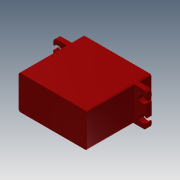
# Autodesk Inventor part: standart_servo
Saved by Autodesk Inventor 2015 (Build 190159000, 159)
## iProperties
Created: 2013-01-22
Part Number: standart_servo
Material: Generic
Document SubType Name: Modeling
Designer: idle-rug
Density: 1 g/cm^3
Appearance: Default
Author: idle-rug
Autodesk Inventor part; units mm, degrees
ref_plane "YZ Plane" through (0, 0, 0) normal (1, 0, 0) x (0, 1, 0)
ref_plane "XZ Plane" through (0, 0, 0) normal (0, 1, 0) x (-1, 0, 0)
ref_plane "XY Plane" through (0, 0, 0) normal (0, 0, 1) x (1, 0, 0)
sketch "Sketch1" plane through (0, 0, 0) normal (0, 1, 0) x (-1, 0, 0)
  line L0 (-20.1, -10) -> (20.1, -10)
  line L1 (20.1, -10) -> (20.1, 10)
  line L2 (20.1, 10) -> (-20.1, 10)
  line L3 (-20.1, 10) -> (-20.1, -10)
  line L4 (-20.1, -10) -> (20.1, 10) construction
  line L5 (20.1, -10) -> (-20.1, 10) construction
  point P0 (0, 0)
  constraints: 12 end point, 2 midpoint, 2 parallel, 1 horizontal, 1 perpendicular
extrude "Extrusion1" add sketch "Sketch1" along normal blind 43.7
sketch "Sketch2" plane through (20.1, 0, 10) normal (1, 0, 0) x (0, 0, -1)
  line L0 (20, 0) -> (20, 43.7) projected
  line L1 (0, 0) -> (0, 43.7) projected
  line L2 (20, 27.8) -> (0, 27.8)
  line L3 (0, 27.8) -> (0, 30.6)
  line L4 (0, 30.6) -> (20, 30.6)
  line L5 (20, 30.6) -> (20, 27.8)
  point P0 (10, 0)
  constraints: 8 end point, 4 point on line, 2 perpendicular, 1 collinear
sketch "Sketch3" plane through (-20.1, 0, -10) normal (-1, 0, 0) x (0, 0, 1)
  line L0 (20, 0) -> (20, 43.7) projected
  line L1 (0, 0) -> (0, 43.7) projected
  line L2 (20, 27.8) -> (0, 27.8)
  line L3 (0, 27.8) -> (0, 30.6)
  line L4 (0, 30.6) -> (20, 30.6)
  line L5 (20, 30.6) -> (20, 27.8)
  point P0 (10, 0)
  constraints: 8 end point, 4 point on line, 2 perpendicular
extrude "Extrusion2" add sketch "Sketch3" along normal blind 7.4
extrude "Extrusion3" add sketch "Sketch2" along normal blind 7.4
sketch "Sketch4" plane through (0, 43.7, 0) normal (0, 1, 0) x (1, 0, 0)
  line L0 (20.1, 10) -> (-20.1, 10) projected
  line L1 (-20.1, 10) -> (-20.1, -10) projected
  line L2 (-20.1, -10) -> (20.1, -10) projected
  line L3 (20.1, -10) -> (20.1, 10) projected
  circle A0 centre (-9.4, 0) radius 6.8
  circle A1 centre (-9.4, 0) radius 5.1
  circle A2 centre (-9.4, 0) radius 3
  constraints: 3 centre point, 2 coincident
extrude "Extrusion4" cut sketch "Sketch4" against normal blind 5.8 contours L3 L2 L1 L0
sketch "Sketch5" plane through (-9.4, 43.7, 0) normal (0, 1, 0) x (1, 0, 0)
  circle A0 centre (0, 0) radius 6.8 projected
  circle A1 centre (0, 0) radius 2.5
  dimension "d20" = 5
  constraints: 1 centre point, 1 coincident
  measures "d20" diameter of A1
extrude "Extrusion5" cut sketch "Sketch5" against normal blind 4
fillet "Fillet1" radius 2 1 edges at (-27.5, 29.2, 10)
fillet "Fillet2" radius 2 1 edges at (27.5, 29.2, 10)
fillet "Fillet3" radius 2 1 edges at (27.5, 29.2, -10)
fillet "Fillet4" radius 2 1 edges at (-27.5, 29.2, -10)
fillet "Fillet5" radius 1 1 edges at (-20.1, 34.25, -10)
fillet "Fillet6" radius 1 1 edges at (-20.1, 13.9, -10)
fillet "Fillet7" radius 1 1 edges at (-20.1, 34.25, 10)
fillet "Fillet8" radius 1 1 edges at (-20.1, 13.9, 10)
fillet "Fillet9" radius 1 1 edges at (20.1, 34.25, 10)
fillet "Fillet10" radius 1 1 edges at (20.1, 13.9, 10)
fillet "Fillet11" radius 1 1 edges at (20.1, 34.25, -10)
fillet "Fillet12" radius 1 1 edges at (20.1, 13.9, -10)
sketch "Sketch6" plane through (-9.4, 43.7, 0) normal (0, 1, 0) x (1, 0, 0)
  circle A0 centre (0, 0) radius 3
  point P0 (9.4, 0)
  constraints: 1 centre point
extrude "Extrusion6" add sketch "Sketch6" against normal blind 4
chamfer "Chamfer3" distance 1.8 distance2 1.6 1 edges at (-16.2, 39.7, 0) measured on face at (-2.6881, 38.5, 1.0908)
sketch "Sketch7" plane through (27.5, 30.6, 8) normal (0, 1, 0) x (1, 0, 0)
  circle A0 centre (-2.65, 12.95) radius 2.35
  circle A1 centre (-2.65, 3.05) radius 2.35
  line L0 (-0.0003, 1.8) -> (-0.66, 1.8)
  line L1 (-0.0003, 4.222) -> (-0.6131, 4.222)
  line L2 (-0.0003, 12.95) -> (-0.0003, 14.2)
  line L3 (-0.0003, 14.2) -> (-0.66, 14.2)
  line L4 (-0.0003, 12.95) -> (-0.0003, 11.7)
  line L5 (-0.0003, 11.7) -> (-0.66, 11.7)
  line L6 (-0.0003, 4.222) -> (-0.0003, 1.8)
  line L7 (0, 16) -> (0, 0) projected
  line L8 (-0.0003, 14.2) -> (2.6929, 14.2)
  line L9 (-0.0003, 11.7) -> (2.6929, 11.7)
  line L10 (2.6929, 11.7) -> (2.6929, 14.2)
  line L11 (-0.0003, 4.222) -> (2.459, 4.222)
  line L12 (-0.0003, 1.8) -> (2.459, 1.8)
  line L13 (2.459, 1.8) -> (2.459, 4.222)
  point P0 (-27.5, 8)
  constraints: 26 end point, 8 perpendicular, 4 point on circle, 2 centre point, 2 parallel
sketch "Sketch8" plane through (-27.5, 30.6, 8) normal (0, 1, 0) x (1, 0, 0)
  circle A0 centre (2.65, 12.95) radius 2.35
  circle A1 centre (2.65, 3.05) radius 2.35
  line L0 (0, 3.05) -> (0, 4.3)
  line L1 (0, 4.3) -> (0, 1.8)
  line L2 (0, 4.3) -> (0.66, 4.3)
  line L3 (0, 1.8) -> (0.66, 1.8)
  line L4 (0, 12.95) -> (0, 11.7)
  line L5 (0, 11.7) -> (0.66, 11.7)
  line L6 (0, 12.95) -> (0, 14.2)
  line L7 (0, 14.2) -> (0.66, 14.2)
  point P0 (27.5, 8)
  constraints: 16 end point, 4 point on circle, 2 centre point, 1 parallel, 1 perpendicular
extrude "Extrusion7" cut sketch "Sketch7" against normal blind 3
extrude "Extrusion8" cut sketch "Sketch8" against normal blind 3
body "Solid1"
